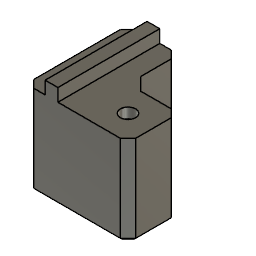
right corner leg (Autodesk Fusion 360 design; units mm, degrees)
Autodesk Fusion 360 part; units mm, degrees
sketch "Szkic1" plane through (0, 0, 0) normal (0, 0, 1) x (1, 0, 0)
  line L0 (0, 0) -> (20, 0)
  line L1 (20, 0) -> (20, -20)
  line L2 (20, -20) -> (0, -20)
  line L3 (0, -20) -> (0, 0)
  line L4 (20, 0) -> (40, 0)
  line L5 (40, 0) -> (40, -20)
  line L6 (40, -20) -> (20, -20)
  line L7 (20, -20) -> (20, 0)
  line L8 (0, 0) -> (0, 20)
  line L9 (0, 20) -> (20, 20)
  line L10 (20, 20) -> (20, 0)
  line L11 (20, 0) -> (0, 0)
  circle A0 centre (30, -10) radius 3
  circle A1 centre (10, 10) radius 3
  line L12 (7.5, 20) -> (12.5, 20)
  line L13 (12.5, 20) -> (12.5, -20)
  line L14 (12.5, -20) -> (7.5, -20)
  line L15 (7.5, -20) -> (7.5, 20)
  line L16 (22.5, -7.5) -> (22.5, -12.5)
  line L17 (40, -12.5) -> (40, -7.5)
  line L18 (40, -7.5) -> (31.6583, -7.5)
  line L19 (28.3417, -7.5) -> (22.5, -7.5)
  line L20 (22.5, -12.5) -> (28.3417, -12.5)
  line L21 (31.6583, -12.5) -> (40, -12.5)
  dimension "d1" = 6
  dimension "d2" = 6
  constraint perpendicular L0 L1
  constraint parallel L0 L2
  constraint parallel L1 L3
  constraint horizontal L0
  constraint coincident L0.start L3.end
  constraint perpendicular L4 L5
  constraint parallel L4 L6
  constraint parallel L5 L7
  constraint perpendicular L1 L4
  constraint perpendicular L8 L9
  constraint parallel L8 L10
  constraint parallel L9 L11
  constraint perpendicular L0 L8
  constraint perpendicular L12 L13
  constraint parallel L12 L14
  constraint parallel L13 L15
  constraint coincident L9 L12.end
  constraint coincident L9 L12.start
  constraint perpendicular L16 L20
  constraint parallel L16 L17
  constraint parallel L18 L21
  constraint vertical L16
  constraint coincident A0 L18.end
  constraint coincident A0 L19.start
  constraint collinear L18 L19
  constraint coincident A0 L20.end
  constraint coincident A0 L21.start
  constraint collinear L20 L21
  measures "d1" diameter of A0
  measures "d2" diameter of A1
extrude "Wyciągnięcie proste1" add sketch "Szkic1" against normal blind 25 contours L0 L8 L9 L11 A1 L15 | L0 L2 L3 L11 L15 | L0 L9 L10 L11 A1 L13 | L0 L1 L2 L7 L11 L13 | A1 L15 | L1 L4 L5 L6 L7 A0 L16 L18 L19 L20 L21 | A1 L13 | L5 A0 L17 L18 L21 | A0 L16 L19 L20 makes body 1 at (7.5, -6.6667, -8.3333) makes body 2 at (12.5, 6.6667, -8.3333)
extrude "Wyciągnięcie proste2" add sketch "Szkic1" against normal blind 25 contours L0 L11 A1 L13 L15 | L0 L2 L11 L13 L14 L15 | A1 L13 L15 | L9 A1 L12 L13 L15 bodies 1 2
extrude "Wyciągnięcie proste3" add sketch "Szkic1" along normal blind 5 contours L0 L11 A1 L13 L15 | L0 L2 L11 L13 L14 L15 | A1 L13 L15 | L9 A1 L12 L13 L15 bodies 1
sketch "Szkic2" plane through (0, 0, -25) normal (0, 0, -1) x (1, 0, 0)
  circle A0 centre (30, 10) radius 3
  line L0 (40, 20) -> (0, 20)
  line L1 (0, 20) -> (0, -20)
  line L2 (0, -20) -> (20, -20)
  line L3 (20, -20) -> (20, 0)
  line L4 (20, 0) -> (40, 0)
  line L5 (40, 0) -> (40, 20)
  circle A1 centre (30, 10) radius 5.5
  dimension "d9" = 11
  constraint concentric A0 A1
  measures "d9" diameter of A1
extrude "Wyciągnięcie proste4" add sketch "Szkic2" against normal blind 21 contours A0 | A1 bodies 1
extrude "Wyciągnięcie proste5" cut sketch "Szkic2" against normal blind 20.8 contours A0 | A1 bodies 1
chamfer "Fazowanie1" distance 3 angle 45 1 edges at (0, 20, -12.5) tangent chain off on bodies 1
chamfer "Fazowanie2" distance 3 angle 45 2 edges at (40, -20, -12.5) (0, -20, -12.5) tangent chain off on bodies 1
chamfer "Fazowanie3" distance 5 angle 45 1 edges at (20, 0, -12.5) tangent chain off on bodies 1
chamfer "Fazowanie4" distance 3 angle 45 2 edges at (40, 0, -12.5) (20, 20, -12.5) tangent chain off on bodies 1
chamfer "Fazowanie5" distance 1 angle 45 1 faces at (6.6667, 1.6667, -25) tangent chain off on bodies 1
delete_face "Usuń powierzchnię1" 1 faces at (36.159, -9.6926, -24.6667) on bodies 1
delete_face "Usuń powierzchnię2" 1 faces at (1.3333, 17.8619, -24.3333) on bodies 1
delete_face "Usuń powierzchnię3" 1 faces at (7.1953, 19.3333, -24.6667) on bodies 1
delete_face "Usuń powierzchnię4" 1 faces at (17.1953, 18.8619, -24.6667) on bodies 1
delete_face "Usuń powierzchnię5" 1 faces at (19.3333, 13.1953, -24.6667) on bodies 1
delete_face "Usuń powierzchnię6" 1 faces at (0.6667, 6.1381, -24.6667) on bodies 1
delete_face "Usuń powierzchnię7" 1 faces at (21.6667, 2.8619, -24.3333) on bodies 1
delete_face "Usuń powierzchnię8" 1 faces at (29.3333, -0.3333, -24.3333) on bodies 1
delete_face "Usuń powierzchnię9" 1 faces at (37.1953, -1.1381, -24.6667) on bodies 1
delete_face "Usuń powierzchnię10" 1 faces at (39.3333, -7.1953, -24.6667) on bodies 1
delete_face "Usuń powierzchnię11" 1 faces at (38.8619, -17.1953, -24.6667) on bodies 1
delete_face "Usuń powierzchnię12" 1 faces at (17.9714, -19.3333, -24.6667) on bodies 1
delete_face "Usuń powierzchnię13" 1 faces at (1.4714, -17.5286, -24.6667) on bodies 1
extrude "Wyciągnięcie proste6" add 1 faces at (6.6667, 1.6667, -25) along direction (0, 0, -1) blind 10 on bodies 1 bodies 1
chamfer "Fazowanie6" distance 1 angle 45 1 faces at (6.6667, 1.6667, -35) tangent chain off on bodies 1
delete_face "Usuń powierzchnię14" 1 faces at (36.159, -10.3074, -34.6667) on bodies 1
